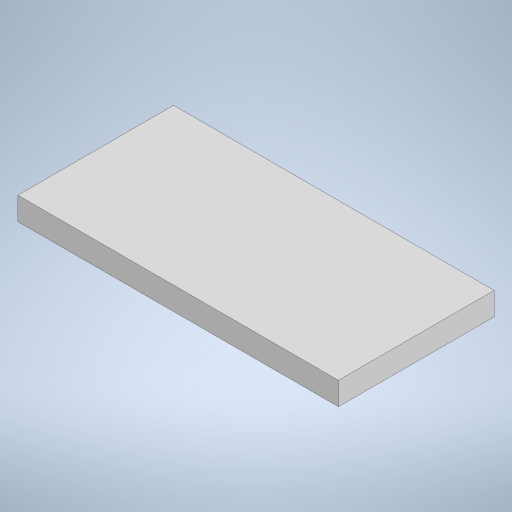
# Autodesk Inventor part: sguard
Saved by Autodesk Inventor 2023 (Build 270158000, 158)
## iProperties
Created: 2023-03-16
Part Number: sguard
Material: Generic
Document SubType Name: Modeling
Designer: ianjo
Density: 1 g/cm^3
Appearance: Default
Author: ianjo
Autodesk Inventor part; units mm, degrees
ref_plane "YZ Plane" through (0, 0, 0) normal (1, 0, 0) x (0, 1, 0)
ref_plane "XZ Plane" through (0, 0, 0) normal (0, 1, 0) x (-1, 0, 0)
ref_plane "XY Plane" through (0, 0, 0) normal (0, 0, 1) x (1, 0, 0)
sketch "Sketch1" plane through (0, 0, 0) normal (0, 1, 0) x (-1, 0, 0)
  line L0 (-44.45, 21.59) -> (44.45, 21.59)
  line L1 (44.45, 21.59) -> (44.45, -21.59)
  line L2 (44.45, -21.59) -> (-44.45, -21.59)
  line L3 (-44.45, -21.59) -> (-44.45, 21.59)
  line L4 (-44.45, 21.59) -> (44.45, -21.59) construction
  line L5 (44.45, 21.59) -> (-44.45, -21.59) construction
  point P0 (0, 0)
  dimension "d5" = 88.9
  dimension "d6" = 43.18
  constraints: 12 end point, 2 midpoint, 2 parallel, 1 horizontal, 1 perpendicular
  measures "d5" distance of L1.end L2.end
  measures "d6" distance of L0.end L1.end
extrude "Extrusion1" add sketch "Sketch1" along normal blind 6.35
body "Solid1"
